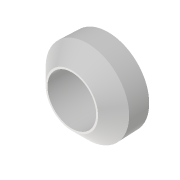
# Autodesk Inventor part: Matchboxscope_M12_Lensadapter_v0
Saved by Autodesk Inventor 2022 (Build 260153000, 153)
## iProperties
Created: 2022-06-17
Part Number: Matchboxscope_M12_Lensadapter_v0
Material: Generisch
Document SubType Name: Modeling
Designer: diederichbenedict
Density: 1 g/cm^3
Appearance: Vorgabe
Author: diederichbenedict
Autodesk Inventor part; units mm, degrees
ref_plane "YZ Plane" through (0, 0, 0) normal (1, 0, 0) x (0, 1, 0)
ref_plane "XZ Plane" through (0, 0, 0) normal (0, 1, 0) x (-1, 0, 0)
ref_plane "XY Plane" through (0, 0, 0) normal (0, 0, 1) x (1, 0, 0)
sketch "Skizze1" plane through (0, 0, 0) normal (1, 0, 0) x (0, 1, 0)
  line L0 (3.35, 3.5525) -> (3.35, -1.7616)
  line L1 (3.35, -1.7616) -> (5.65, -1.7616)
  line L2 (5.65, -1.7616) -> (5.75, 1.0958)
  line L3 (5.75, 1.0958) -> (3.6074, 3.2384)
  line L4 (3.6074, 3.2384) -> (3.35, 3.2384)
  line L5 (0, 3.5525) -> (0, -4.0298)
  point P0 (0, 0)
  dimension "d0" = 3.35
  dimension "d1" = 5.65
  dimension "d2" = 5.75
  dimension "d3" = 5
  dimension "d4" = 45
  constraints: 12 end point, 2 perpendicular, 2 vertical, 1 point on line
  measures "d0" distance from line of point (0, 0) L0
  measures "d1" horizontal distance of point (0, 0) L1.end
  measures "d2" horizontal distance of point (0, 0) L2.end
  measures "d3" distance between parallel lines of L4 L1
  measures "d4" angle of L4 L3
revolve "Umdrehung1" add sketch "Skizze1" angle 360 about axis through (0, 0, 3.5525) along (0, 0, -1)
